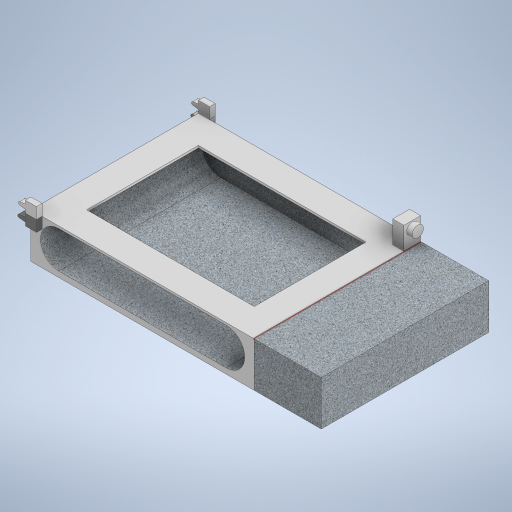
# Autodesk Inventor part: base
Saved by Autodesk Inventor 2023 (Build 270158030, 158C)
## iProperties
Created: 2022-05-25
Part Number: base
Material: Genérico
Document SubType Name: Modeling
Designer: isaac
Density: 1 g/cm^3
Appearance: Valor por defecto
Author: isaac
Autodesk Inventor part; units mm, degrees
ref_plane "YZ Plane" through (0, 0, 0) normal (1, 0, 0) x (0, 1, 0)
ref_plane "XZ Plane" through (0, 0, 0) normal (0, 1, 0) x (-1, 0, 0)
ref_plane "XY Plane" through (0, 0, 0) normal (0, 0, 1) x (1, 0, 0)
sketch "Boceto1" plane through (0, 0, 0) normal (0, 0, 1) x (1, 0, 0)
  point P0 (0, 0)
sketch "Boceto2" plane through (0, 0, 0) normal (0, 0, 1) x (1, 0, 0)
  line L0 (-1000, 200) -> (1000, 200)
  line L1 (1000, 200) -> (1000, -200)
  line L2 (1000, -200) -> (-1000, -200)
  line L3 (-1000, -200) -> (-1000, 200)
  point P0 (0, 0)
  point P1 (1000, 0)
  point P2 (0, 200)
  dimension "d0" = 2000
  dimension "d1" = 400
  constraints: 8 end point, 2 midpoint, 2 parallel, 1 horizontal, 1 horizontal alignment, 1 perpendicular, 1 vertical alignment
  measures "d0" distance between parallel lines of L1 L3
  measures "d1" distance between parallel lines of L2 L0
extrude "Extrusión1" add sketch "Boceto2" along normal blind 1500
sketch "Boceto3" plane through (-1000, 200, 0) normal (0, 1, 0) x (1, 0, 0)
  line L0 (2000, 0) -> (0, 0) construction
  line L1 (0, 0) -> (0, -1500) construction
  line L2 (2000, -1500) -> (0, -1500) construction
  line L3 (2000, 0) -> (2000, -1500) construction
  line L4 (1750, -1250) -> (250, -1250)
  line L5 (250, -1250) -> (250, -250)
  line L6 (250, -250) -> (1750, -250)
  line L7 (1750, -250) -> (1750, -1250)
  point P0 (1000, 0)
  point P1 (1750, -750)
  dimension "d4" = 1500
  constraints: 8 end point, 1 midpoint, 3 other
  measures "d4" distance from line of point (1750, -750) L5
extrude "Extrusión2" cut sketch "Boceto3" against normal blind 350
sketch "Boceto4" plane through (0, 0, 1500) normal (0, 0, 1) x (1, 0, 0)
  line L0 (750, 200) -> (-750, 200) construction
  line L1 (750, 200) -> (750, -150) construction
  line L2 (750, -150) -> (-750, -150) construction
  line L3 (-750, 200) -> (-750, -150) construction
  line L4 (-750, 200) -> (-750, -150) projected
  line L5 (-750, -150) -> (750, -150) projected
  line L6 (-750, 180) -> (750, 180)
  line L7 (750, -150) -> (-750, -150)
  line L8 (750, 200) -> (750, -150) projected
  arc A0 (750, -150) -> (750, 180) centre (750, 15) ccw
  arc A1 (-750, 180) -> (-750, -150) centre (-750, 15) ccw
  point P0 (0, 0)
  dimension "d7" = 20
  dimension "d8" = 165
  constraints: 4 end point, 4 point on circle, 3 tangent, 2 centre point, 1 horizontal, 1 parallel, 1 point on line
  measures "d7" distance between parallel lines of L6 L0
  measures "d8" radius of A0
extrude "Extrusión3" cut sketch "Boceto4" against normal blind 1450
sketch "Boceto5" plane through (1000, -200, 0) normal (1, 0, 0) x (0, 0, -1)
  line L0 (0, 0) -> (0, 400) construction
  line L1 (0, 400) -> (-1500, 400) construction
  line L2 (-1500, 0) -> (-1500, 400) construction
  line L3 (0, 0) -> (-1500, 0) construction
  line L4 (0, 400) -> (-1500, 400) projected
  line L5 (-1500, 400) -> (0, 400)
  line L6 (0, 400) -> (0, 0)
  line L7 (0, 0) -> (-1500, 0)
  line L8 (-1500, 0) -> (-1500, 400)
  point P0 (0, 200)
  constraints: 8 end point, 2 parallel, 1 horizontal, 1 perpendicular
extrude "Extrusión4" add sketch "Boceto5" along normal blind 600 separate body
sketch "Boceto6" plane through (-1000, 200, 0) normal (0, 1, 0) x (1, 0, 0)
  line L0 (250, -1250) -> (250, -250) construction
  line L1 (250, -250) -> (1750, -250) construction
  line L2 (1750, -250) -> (1750, -1250) construction
  line L3 (1750, -1250) -> (250, -1250) construction
  line L4 (2000, 0) -> (0, 0) construction
  line L5 (0, 0) -> (0, -1500) construction
  line L6 (2000, -1500) -> (0, -1500) construction
  line L7 (2000, 0) -> (2000, -1500) construction
  line L8 (0, 0) -> (2000, 0) projected
  line L9 (1990, 0) -> (1890, 0)
  line L10 (1890, 0) -> (1890, -150)
  line L11 (1890, -150) -> (1990, -150)
  line L12 (1990, -150) -> (1990, 0)
  point P0 (1000, 0)
  point P1 (1890, 0)
  dimension "d13" = 150
  dimension "d14" = 100
  dimension "d15" = 10
  constraints: 8 end point, 2 parallel, 1 horizontal, 1 perpendicular, 1 point on line
  measures "d13" distance between parallel lines of L4 L11
  measures "d14" distance between parallel lines of L12 L10
  measures "d15" distance between parallel lines of L7 L12
extrude "Extrusión5" add sketch "Boceto6" along normal blind 200 separate body
sketch "Boceto7" plane through (990, 200, 150) normal (1, 0, 0) x (0, 0, -1)
  line L0 (0, 0) -> (150, 0) construction
  line L1 (150, 0) -> (150, 200) construction
  line L2 (0, 200) -> (150, 200) construction
  line L3 (0, 0) -> (0, 200) construction
  circle A0 centre (75, 140) radius 50
  line L4 (0, 200) -> (150, 200) projected
  point P0 (150, -200)
  point P1 (75, 200)
  point P2 (75, 200)
  dimension "d18" = 100
  dimension "d19" = 60
  constraints: 2 midpoint, 1 centre point, 1 vertical alignment
  measures "d18" diameter of A0
  measures "d19" distance of A0.centre point (75, 200)
extrude "Extrusión6" add sketch "Boceto7" along normal blind 50 separate body
sketch "Boceto8" plane through (0, 0, 1500) normal (0, 0, 1) x (1, 0, 0)
  line L0 (750, -150) -> (-750, -150) construction
  arc A0 (-750, 180) -> (-750, -150) centre (-750, 15) ccw construction
  line L1 (-750, 180) -> (750, 180) construction
  arc A1 (750, -150) -> (750, 180) centre (750, 15) ccw construction
  line L2 (-1000, -200) -> (1000, -200) construction
  line L3 (1000, -200) -> (1000, 200) construction
  line L4 (1000, 200) -> (-1000, 200) construction
  line L5 (-1000, 200) -> (-1000, -200) construction
  line L6 (1000, 200) -> (1000, -200) construction
  line L7 (1000, -200) -> (1600, -200) construction
  line L8 (1600, 200) -> (1600, -200) construction
  line L9 (1000, 200) -> (1600, 200) construction
  line L10 (1000, 200) -> (-1000, 200) projected
  line L11 (992, 200) -> (1022, 200)
  line L12 (1000, 200) -> (1600, 200) projected
  arc A2 (992, 200) -> (1022, 200) centre (1007, 200) ccw
  line L13 (890, 200) -> (990, 200) construction
  line L14 (990, 200) -> (990, 400) construction
  line L15 (890, 400) -> (990, 400) construction
  line L16 (890, 200) -> (890, 400) construction
  point P0 (0, 0)
  dimension "d22" = 30
  dimension "d24" = 2
  constraints: 2 end point, 2 point on circle, 2 point on line, 1 centre point, 1 midpoint
  measures "d22" distance of L11.start L11.end
  measures "d24" distance from line of L11.start L14
extrude "Extrusión7" cut sketch "Boceto8" against normal through all bodies 1
sketch "Boceto9" plane through (0, 0, 1500) normal (0, 0, 1) x (1, 0, 0)
  arc A0 (992, 200) -> (1000, 186.7335) centre (1007, 200) ccw construction
  line L0 (992, 200) -> (-1000, 200) construction
  line L1 (-1000, 200) -> (-1000, -200) construction
  line L2 (-1000, -200) -> (1000, -200) construction
  line L3 (1000, -200) -> (1000, 186.7335) construction
  line L4 (750, -150) -> (-750, -150) construction
  arc A1 (-750, 180) -> (-750, -150) centre (-750, 15) ccw construction
  line L5 (-750, 180) -> (750, 180) construction
  arc A2 (750, -150) -> (750, 180) centre (750, 15) ccw construction
  line L6 (-1000, 200) -> (-1000, -200) projected
  line L7 (-1000, 200) -> (-900, 200)
  line L8 (-900, 200) -> (-900, 100)
  line L9 (-900, 100) -> (-1000, 100)
  line L10 (-1000, 100) -> (-1000, 200)
  point P0 (0, 0)
  dimension "d27" = 100
  dimension "d28" = 100
  constraints: 8 end point, 2 parallel, 1 horizontal, 1 perpendicular
  measures "d27" distance between parallel lines of L9 L0
  measures "d28" distance between parallel lines of L1 L8
extrude "Extrusión8" add sketch "Boceto9" along normal blind 50 separate body
sketch "Boceto10" plane through (0, 0, 0) normal (0, 0, -1) x (-1, 0, 0)
  arc A0 (-1000, 186.7335) -> (-992, 200) centre (-1007, 200) ccw construction
  line L0 (-1000, -200) -> (-1000, 186.7335) construction
  line L1 (1000, -200) -> (-1000, -200) construction
  line L2 (1000, 200) -> (1000, -200) construction
  line L3 (-992, 200) -> (1000, 200) construction
  line L4 (1000, 200) -> (900, 200)
  line L5 (900, 200) -> (900, 100)
  line L6 (900, 100) -> (1000, 100)
  line L7 (1000, 100) -> (1000, 200)
  point P0 (0, 0)
  dimension "d31" = 100
  dimension "d32" = 100
  constraints: 8 end point, 2 parallel, 1 horizontal, 1 perpendicular
  measures "d31" distance of L6.end L5.end
  measures "d32" distance of L5.end L4.end
extrude "Extrusión9" add sketch "Boceto10" along normal blind 50 separate body
sketch "Boceto11" plane through (0, 0, -50) normal (0, 0, -1) x (-1, 0, 0)
  line L0 (900, 200) -> (900, 100) construction
  line L1 (900, 100) -> (1000, 100) construction
  line L2 (1000, 100) -> (1000, 200) construction
  line L3 (1000, 200) -> (900, 200) construction
  circle A0 centre (1054.5004, 150) radius 50 construction
  line L4 (1000, 200) -> (1000, -200) construction
  line L5 (1000, 150) -> (1000, 170) construction
  circle A1 centre (1054.5004, 150) radius 14.1882 construction
  line L6 (1000, 150) -> (1000, 170)
  line L7 (1000, 170) -> (1055.9849, 164.1103)
  line L8 (1000, 150) -> (1000, 130)
  line L9 (1000, 130) -> (1054.5004, 135.8118)
  arc A2 (1054.5004, 135.8118) -> (1055.9849, 164.1103) centre (1054.5004, 150) ccw
  point P0 (0, 0)
  dimension "d35" = 100
  dimension "d36" = 20
  dimension "d37" = 20
  constraints: 10 end point, 4 point on circle, 3 centre point, 3 point on line, 2 tangent, 1 collinear
  measures "d35" diameter of A0
  measures "d36" distance of L5.start L5.end
  measures "d37" distance of L5.start L8.end
extrude "Extrusión10" add sketch "Boceto11" against normal blind 50 separate body
sketch "Boceto12" plane through (0, 0, 1550) normal (0, 0, 1) x (1, 0, 0)
  line L0 (-900, 200) -> (-1000, 200) construction
  line L1 (-1000, 200) -> (-1000, 100) construction
  line L2 (-1000, 100) -> (-900, 100) construction
  line L3 (-900, 100) -> (-900, 200) construction
  arc A0 (-1055.9849, 164.1103) -> (-1054.5004, 135.8118) centre (-1054.5004, 150) ccw construction
  line L4 (-1054.5004, 135.8118) -> (-1000, 130) construction
  line L5 (-1000, 130) -> (-1000, 170) construction
  line L6 (-1000, 170) -> (-1055.9849, 164.1103) construction
  line L7 (-1000, 130) -> (-1000, 170)
  line L8 (-1000, 200) -> (-1000, -200) projected
  line L9 (-1000, 170) -> (-1055.9849, 164.1103) projected
  line L10 (-1000, 170) -> (-1055.9849, 164.1103)
  arc A1 (-1055.9849, 164.1103) -> (-1054.5004, 135.8118) centre (-1054.5004, 150) ccw
  line L11 (-1054.5004, 135.8118) -> (-1000, 130)
  point P0 (0, 0)
  constraints: 6 end point, 2 collinear, 2 point on circle, 2 tangent, 1 centre point
extrude "Extrusión11" add sketch "Boceto12" against normal blind 50 separate body
sketch "Boceto13" plane through (0, 0, 1550) normal (0, 0, 1) x (1, 0, 0)
  line L0 (-900, 200) -> (-1000, 200) construction
  line L1 (-1000, 200) -> (-1000, 100) construction
  line L2 (-1000, 100) -> (-900, 100) construction
  line L3 (-900, 100) -> (-900, 200) construction
  line L4 (-1000, 200) -> (-1000, -200) projected
  line L5 (-1000, 200) -> (-900, 200)
  line L6 (-900, 200) -> (-900, 300)
  line L7 (-900, 300) -> (-1000, 300)
  line L8 (-1000, 300) -> (-1000, 200)
  circle A0 centre (-1050, 250) radius 50 construction
  circle A1 centre (-1050, 250) radius 14.188 construction
  line L9 (-1000, 250) -> (-1000, 270)
  line L10 (-1000, 270) -> (-1050, 264.188)
  arc A2 (-1050, 264.188) -> (-1046.7455, 236.1903) centre (-1048.3728, 250.1891) ccw
  line L11 (-1000, 250) -> (-1000, 230)
  line L12 (-1000, 230) -> (-1046.7455, 236.1903)
  point P0 (0, 0)
  dimension "d50" = 100
  dimension "d48" = 100
  dimension "d49" = 100
  dimension "d51" = 28.376
  dimension "d52" = 20
  dimension "d53" = 20
  dimension "d54" = 50
  dimension "d55" = 46.7456
  constraints: 16 end point, 4 point on circle, 2 centre point, 2 horizontal alignment, 2 midpoint, 2 parallel, 2 point on line, 1 horizontal, 1 perpendicular, 1 tangent, 1 vertical, 2 other
  measures "d48" distance of L7.end L6.end
  measures "d49" distance of L6.end L5.end
  measures "d51" diameter of A1
  measures "d52" distance of L9.start L9.end
  measures "d53" distance of L9.start L11.end
  measures "d54" horizontal distance of L9.end L10.end
  measures "d55" horizontal distance of L11.end L12.end
extrude "Extrusión12" add sketch "Boceto13" against normal blind 50 separate body
sketch "Boceto14" plane through (0, 0, -50) normal (0, 0, -1) x (-1, 0, 0)
  line L0 (1000, 270) -> (1000, 300) construction
  line L1 (1000, 300) -> (900, 300) construction
  line L2 (900, 300) -> (900, 200) construction
  line L3 (900, 200) -> (1000, 200) construction
  line L4 (1000, 200) -> (1000, 230) construction
  line L5 (1000, 230) -> (1046.7455, 236.1903) construction
  arc A0 (1046.7455, 236.1903) -> (1050, 264.188) centre (1048.3728, 250.1891) ccw construction
  line L6 (1050, 264.188) -> (1000, 270) construction
  line L7 (1000, 270) -> (1000, 300) projected
  line L8 (1000, 270) -> (1000, 300)
  line L9 (1000, 300) -> (900, 300) projected
  line L10 (1000, 300) -> (900, 300)
  line L11 (900, 300) -> (900, 200)
  line L12 (-992, 200) -> (1000, 200) construction
  line L13 (900, 200) -> (1000, 200)
  line L14 (1000, 200) -> (1000, 230) projected
  line L15 (1000, 200) -> (1000, 230)
  line L16 (1000, 230) -> (1050.1043, 236.2028)
  arc A1 (1050.1043, 236.2028) -> (1050, 264.188) centre (1048.3728, 250.1891) ccw
  line L17 (1050, 264.188) -> (1000, 270) projected
  line L18 (1050, 264.188) -> (1000, 270)
  point P0 (0, 0)
  constraints: 14 end point, 4 collinear, 3 point on circle, 3 tangent, 2 perpendicular, 1 centre point
extrude "Extrusión13" add sketch "Boceto14" against normal blind 50 separate body
sketch "Boceto15" plane through (0, 0, 0) normal (1, 0, 0) x (0, 1, 0)
  point P0 (0, 0)
